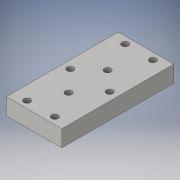
# Autodesk Inventor part: ROV Motor plate
Saved by Autodesk Inventor 2016 (Build 200138000, 138)
## iProperties
Created: 2017-03-09
Part Number: ROV Motor plate
Material: Generic
Document SubType Name: Modeling
Designer: Student
Density: 1 g/cm^3
Appearance: Default
Author: Student
Autodesk Inventor part; units mm, degrees
ref_plane "YZ Plane" through (0, 0, 0) normal (1, 0, 0) x (0, 1, 0)
ref_plane "XZ Plane" through (0, 0, 0) normal (0, 1, 0) x (-1, 0, 0)
ref_plane "XY Plane" through (0, 0, 0) normal (0, 0, 1) x (1, 0, 0)
sketch "Sketch1" plane through (0, 0, 0) normal (0, 1, 0) x (-1, 0, 0)
  line L0 (0, 0) -> (-25.4, 0)
  line L1 (-25.4, 0) -> (-25.4, -51.2064)
  line L2 (-25.4, -51.2064) -> (0, -51.2064)
  line L3 (0, -51.2064) -> (0, 0)
  dimension "d0" = 25.4
  dimension "d1" = 51.2064
  constraints: 8 end point, 2 parallel, 1 horizontal, 1 perpendicular
  measures "d0" distance of L2.end L1.end
  measures "d1" distance of L1.end L0.end
extrude "Extrusion1" add sketch "Sketch1" along normal blind 7.62
sketch "Sketch2" plane through (0, 7.62, 0) normal (0, 1, 0) x (1, 0, 0)
  line L0 (25.4, 51.2064) -> (0, 51.2064) projected
  line L1 (0, 0) -> (25.4, 0) projected
  line L2 (0, 51.2064) -> (0, 0) projected
  line L3 (25.4, 0) -> (25.4, 51.2064) projected
  point P0 (6.35, 48.0314)
  point P1 (19.05, 48.0314)
  point P2 (19.05, 3.175)
  point P3 (6.35, 3.175)
  dimension "d4" = 3.175
  dimension "d5" = 3.175
  dimension "d6" = 3.175
  dimension "d7" = 3.175
  dimension "d8" = 6.35
  dimension "d9" = 6.35
  dimension "d10" = 6.35
  dimension "d11" = 6.35
  measures "d4" distance from line of point (6.35, 48.031) L0
  measures "d5" distance from line of L0 point (19.05, 48.031)
  measures "d6" distance from line of L1 point (6.35, 3.175)
  measures "d7" distance from line of L1 point (19.05, 3.175)
  measures "d8" distance from line of L2 point (6.35, 3.175)
  measures "d9" distance from line of L3 point (19.05, 3.175)
  measures "d10" distance from line of L2 point (6.35, 48.031)
  measures "d11" distance from line of L3 point (19.05, 48.031)
hole "Hole1" at (6.35, 7.62, -48.0314) at (19.05, 7.62, -48.0314) at (19.05, 7.62, -3.175) at (6.35, 7.62, -3.175) direction (0, -1, 0) diameter 3 end through all
sketch "Sketch3" plane through (0, 7.62, 0) normal (0, 1, 0) x (1, 0, 0)
  line L0 (25.4, 0) -> (25.4, 51.2064) projected
  line L1 (25.4, 51.2064) -> (0, 51.2064) projected
  line L2 (12.7, 51.2064) -> (12.7, -5.0328) construction
  point P0 (0, 0)
  point P1 (3.683, 25.6032)
  point P2 (21.717, 25.6032)
  point P3 (12.7, 33.654)
  point P4 (12.7, 15.8232)
  dimension "d26" = 25.6032
  dimension "d27" = 18.034
  dimension "d28" = 17.8308
  constraints: 2 end point, 2 point on line, 1 midpoint, 1 symmetric about line, 1 vertical
  measures "d26" distance from line of point (3.683, 25.603) L1
  measures "d27" distance of point (3.683, 25.603) point (21.717, 25.603)
  measures "d28" distance of point (12.7, 15.823) point (12.7, 33.654)
hole "Hole2" at (3.683, 7.62, -25.6032) at (21.717, 7.62, -25.6032) at (12.7, 7.62, -33.654) at (12.7, 7.62, -15.8232) direction (0, -1, 0) diameter 3 end through all
body "Solid1"
